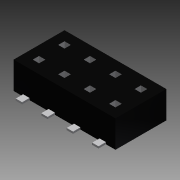
# Autodesk Inventor part: 2mm2Row8PosFemale
Saved by Autodesk Inventor 2014 (Build 180170000, 170)
## iProperties
Created: 2015-11-06
Part Number: 2mm2Row8PosFemale
Material: Generic
Document SubType Name: Modeling
Designer: Owner
Density: 1 g/cm^3
Appearance: Default
Author: Owner
Autodesk Inventor part; units mm, degrees
ref_plane "YZ Plane" through (0, 0, 0) normal (1, 0, 0) x (0, 1, 0)
ref_plane "XZ Plane" through (0, 0, 0) normal (0, 1, 0) x (-1, 0, 0)
ref_plane "XY Plane" through (0, 0, 0) normal (0, 0, 1) x (1, 0, 0)
sketch "Sketch1" plane through (0, 0, 0) normal (0, 1, 0) x (-1, 0, 0)
  line L0 (-6.3636, 1.5475) -> (1.6364, 1.5475)
  line L1 (1.6364, 1.5475) -> (1.6364, -2.4525)
  line L2 (1.6364, -2.4525) -> (-6.3636, -2.4525)
  line L3 (-6.3636, -2.4525) -> (-6.3636, 1.5475)
  point P0 (0, 0)
  dimension "d0" = 4
  dimension "d1" = 8
  constraints: 8 end point, 2 parallel, 1 horizontal, 1 perpendicular
  measures "d0" distance of L0.end L1.end
  measures "d1" distance of L0.start L0.end
extrude "Extrusion1" add sketch "Sketch1" along normal blind 2.13
sketch "Sketch3" plane through (0, 0, 0) normal (0, -1, 0) x (1, 0, 0)
  line L0 (6.3636, 1.5475) -> (-1.6364, 1.5475) projected
  line L1 (-1.6364, 1.5475) -> (-1.6364, -2.4525) projected
  line L2 (-0.8864, 2.1275) -> (-0.3864, 2.1275)
  line L3 (-0.3864, 2.1275) -> (-0.3864, -3.0325)
  line L4 (-0.3864, -3.0325) -> (-0.8864, -3.0325)
  line L5 (-0.8864, -3.0325) -> (-0.8864, 2.1275)
  point P0 (0, 0)
  dimension "d4" = 0.5
  dimension "d5" = 5.16
  dimension "d6" = 0.58
  dimension "d7" = 0.75
  constraints: 8 end point, 2 parallel, 1 horizontal, 1 perpendicular
  measures "d4" distance of L2.start L2.end
  measures "d5" distance of L4.end L2.start
  measures "d6" distance between parallel lines of L0 L2
  measures "d7" distance between parallel lines of L1 L5
extrude "Extrusion2" add sketch "Sketch3" against normal blind 0.15
pattern_linear "Rectangular Pattern1" count 4 spacing 2 along (1, 0, 0) of "Extrusion2"
sketch "Sketch4" plane through (0, 2.13, 0) normal (0, 1, 0) x (1, 0, 0)
  line L0 (6.3636, 2.4525) -> (-1.6364, 2.4525) projected
  line L1 (-1.6364, 2.4525) -> (-1.6364, -1.5475) projected
  line L2 (-0.8864, 1.7025) -> (-0.3864, 1.7025)
  line L3 (-0.3864, 1.7025) -> (-0.3864, 1.2025)
  line L4 (-0.3864, 1.2025) -> (-0.8864, 1.2025)
  line L5 (-0.8864, 1.2025) -> (-0.8864, 1.7025)
  point P0 (0, 0)
  dimension "d13" = 0.5
  dimension "d14" = 0.5
  dimension "d15" = 0.75
  dimension "d16" = 0.75
  constraints: 8 end point, 2 parallel, 1 horizontal, 1 perpendicular
  measures "d13" distance of L2.end L3.end
  measures "d14" distance of L2.start L2.end
  measures "d15" distance between parallel lines of L1 L5
  measures "d16" distance between parallel lines of L0 L2
extrude "Extrusion3" cut sketch "Sketch4" against normal through all
pattern_linear "Rectangular Pattern2" count 4 spacing 2 along (1, 0, 0) count 2 spacing 2 along (0, 0, 1) of "Extrusion3"
body "Solid1"
